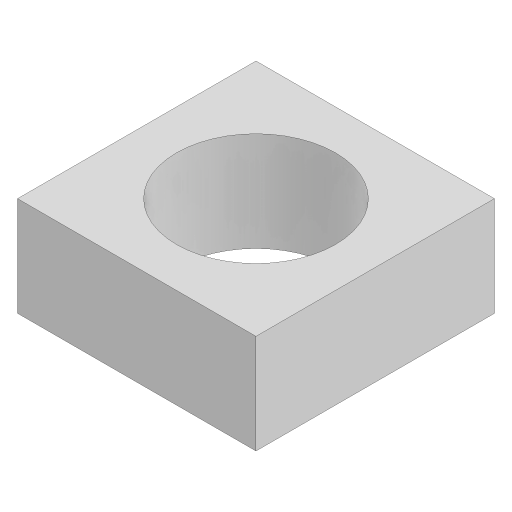
# Autodesk Inventor part: endcap_4mm_2ea_air_inlet
Saved by Autodesk Inventor 2023 (Build 270158000, 158)
## iProperties
Created: 2023-11-06
Part Number: endcap_4mm_2ea_air_inlet
Material: 일반
Document SubType Name: Modeling
Designer: Gihyeok Na
Density: 1 g/cm^3
Appearance: 기본값
Author: Gihyeok Na
Autodesk Inventor part; units mm, degrees
ref_plane "YZ Plane" through (0, 0, 0) normal (1, 0, 0) x (0, 1, 0)
ref_plane "XZ Plane" through (0, 0, 0) normal (0, 1, 0) x (-1, 0, 0)
ref_plane "XY Plane" through (0, 0, 0) normal (0, 0, 1) x (1, 0, 0)
sketch "스케치1" plane through (0, 0, 0) normal (0, 1, 0) x (-1, 0, 0)
  circle A0 centre (0, 0) radius 1.6
  circle A1 centre (0, 0) radius 2.4
  line L0 (2.4, 2.4) -> (-2.4, 2.4)
  line L1 (-2.4, 2.4) -> (-2.4, -2.4)
  line L2 (-2.4, -2.4) -> (2.4, -2.4)
  line L3 (2.4, -2.4) -> (2.4, 2.4)
  point P0 (2.4, 0)
  point P1 (0, -2.4)
  point P2 (0, 2.4)
  point P3 (-2.4, 0)
  dimension "d0" = 3.2
  dimension "d1" = 4.8
  constraints: 8 end point, 4 tangent, 2 centre point, 2 coincident, 2 parallel, 1 horizontal, 1 perpendicular
  measures "d0" diameter of A0
  measures "d1" diameter of A1
extrude "돌출1" add sketch "스케치1" along normal blind 2
